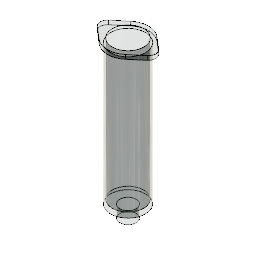
dddd11c0-e493-488c-b1b6-4b4cd47b6b13 (Autodesk Fusion 360 design; units mm, degrees)
Autodesk Fusion 360 part; units mm, degrees
note: some values were not read from the file. Set by a fixed rule: which sketch regions a step uses.
sketch "Sketch3" plane through (0, 0, 0) normal (0, 0, 1) x (1, 0, 0)
  circle A0 centre (0, 0) radius 5.08
  dimension "d5" = 10.16
  constraint coincident A0.centre origin
  measures "d5" diameter of A0
extrude "Extrude2" add sketch "Sketch3" along normal blind 7.62
sketch "Sketch4" plane through (0, 0, 7.62) normal (0, 0, 1) x (-1, 0, 0)
  circle A0 centre (0, 0) radius 5.08
  circle A1 centre (0, 0) radius 10.795
  dimension "d8" = 21.59
  constraint coincident A0.centre A1.centre
  measures "d8" diameter of A1
extrude "Extrude3" add sketch "Sketch4" along normal blind 86.36 contours A0 | A1
sketch "Sketch7" plane through (0, 0, 93.98) normal (0, 0, 1) x (-1, 0, 0)
  circle A0 centre (0, 0) radius 10.795
  circle A1 centre (0, 0) radius 12.7
  circle A2 centre (-12.7, -0.0001) radius 4.5016
  circle A3 centre (12.6996, -0.1003) radius 4.5018
  line L0 (15.5784, -3.5613) -> (8.1213, -9.7639)
  line L1 (-8.1983, -9.6993) -> (-15.606, -3.4381)
  line L2 (-15.606, 3.4379) -> (-8.1984, 9.6993)
  line L3 (8.2745, 9.6344) -> (15.6327, 3.3149)
  circle A4 centre (0, 0) radius 12.7
  dimension "d14" = 25.4
  constraint coincident A0.centre A1.centre
  constraint coincident A1 A2.centre
  constraint coincident A1 A3.centre
  constraint coincident A3 L0.start
  constraint coincident A1 L0.end
  constraint coincident A1 L1.start
  constraint coincident A2 L1.end
  constraint tangent A2 L1
  constraint coincident A2 L2.start
  constraint coincident A1 L2.end
  constraint tangent A1 L2
  constraint coincident A1 L3.start
  constraint coincident A3 L3.end
  constraint tangent A1 L0
  constraint tangent A1 L1
  constraint tangent A3 L0
  constraint tangent A3 L3
  constraint tangent A1 L3
  constraint tangent A2 L2
  constraint coincident A3.centre A4
  measures "d14" diameter of A4
extrude "Extrude4" add sketch "Sketch7" along normal blind 2.54
sketch "Sketch8" plane through (0, 0, 96.52) normal (0, 0, 1) x (-1, 0, 0)
  arc A0 (-15.606, 3.4379) -> (-15.606, -3.4381) centre (-12.7, -0.0001) ccw
  line L0 (-15.606, -3.4381) -> (-8.1983, -9.6993)
  arc A1 (-8.1983, -9.6993) -> (8.1213, -9.7639) centre (0, 0) ccw
  line L1 (8.1213, -9.7639) -> (15.5784, -3.5613)
  arc A2 (15.5784, -3.5613) -> (15.6327, 3.3149) centre (12.6996, -0.1003) ccw
  line L2 (15.6327, 3.3149) -> (8.2745, 9.6344)
  arc A3 (8.2745, 9.6344) -> (-8.1984, 9.6993) centre (0, 0) ccw
  line L3 (-8.1984, 9.6993) -> (-15.606, 3.4379)
  circle A4 centre (0, 0) radius 9.779
  dimension "d15" = 19.558
  constraint coincident A1.centre A3.centre
  measures "d15" diameter of A4
extrude "Extrude5" cut sketch "Sketch8" against normal blind 86.36 contours A4
